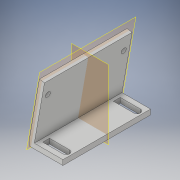
# Autodesk Inventor part: Part2
Saved by Autodesk Inventor 2019 (Build 230136000, 136)
## iProperties
Created: 2019-01-08
Part Number: Part2
Material: Generic
Document SubType Name: Modeling
Designer: Mataria
Density: 1 g/cm^3
Appearance: Default
Author: Mataria
Autodesk Inventor part; units mm, degrees
ref_plane "YZ Plane" through (0, 0, 0) normal (1, 0, 0) x (0, 1, 0)
ref_plane "XZ Plane" through (0, 0, 0) normal (0, 1, 0) x (-1, 0, 0)
ref_plane "XY Plane" through (0, 0, 0) normal (0, 0, 1) x (1, 0, 0)
sketch "Sketch1" plane through (0, 0, 0) normal (1, 0, 0) x (0, 1, 0)
  point P0 (0, 0)
sketch "Sketch2" plane through (0, 0, 0) normal (0, 0, 1) x (1, 0, 0)
  line L0 (0, 0) -> (20, 0)
  line L1 (20, 0) -> (20, 3)
  line L2 (0, 0) -> (0, 3)
  line L3 (0, 3) -> (6.0777, 37.4683)
  line L4 (0, 3) -> (35, 3) construction
  line L5 (6.0777, 37.4683) -> (9.0321, 36.9473)
  line L6 (9.0321, 36.9473) -> (3.0463, 3)
  line L7 (3.0463, 3) -> (20, 3)
  dimension "d0" = 20
  dimension "d1" = 3
  dimension "d2" = 3
  dimension "d4" = 35
  dimension "d5" = 80
  dimension "d6" = 3
  constraints: 16 end point, 2 horizontal, 2 perpendicular, 1 equal length, 1 point on line, 1 vertical
  measures "d0" distance of L0.start L0.end
  measures "d1" distance of L0.end L1.end
  measures "d2" distance of L0.start L2.end
  measures "d4" distance of L2.end L3.end
  measures "d5" angle of L4 L3
  measures "d6" distance of L3.end L5.end
extrude "Extrusion1" add sketch "Sketch2" along normal blind 26 and the other way blind 26
ref_plane "Work Plane1" through (7.5549, 37.2078, 26) normal (0.9848, -0.1736, 0) x (0, 0, -1)
ref_plane "Work Plane2" through (0, 0, 0) normal (0, 0, 1) x (1, 0, 0)
sketch "Sketch3" plane through (9.0321, 36.9473, 26) normal (0.9848, -0.1736, 0) x (0, 0, -1)
  point P0 (26, -37.9544)
sketch "Sketch4" plane through (9.0321, 36.9473, 26) normal (0.9848, -0.1736, 0) x (0, 0, -1)
  circle A0 centre (3.5, -8.527) radius 1.5
  circle A1 centre (48.5, -8.527) radius 1.5
  point P0 (26, -37.9544)
  dimension "d11" = 3
  dimension "d12" = 3
  constraints: 2 centre point
  measures "d11" diameter of A0
  measures "d12" diameter of A1
extrude "Extrusion2" cut sketch "Sketch4" against normal blind 3 contours A0
sketch "Sketch5" plane through (9.0321, 36.9473, 26) normal (0.9848, -0.1736, 0) x (0, 0, -1)
  circle A0 centre (48.5, -8.527) radius 1.5
  point P0 (26, -37.9544)
  dimension "d15" = 3
  constraints: 1 centre point
  measures "d15" diameter of A0
extrude "Extrusion3" cut sketch "Sketch5" against normal blind 3
sketch "Sketch6" plane through (3.0463, 3, 26) normal (0, 1, 0) x (1, 0, 0)
  point P0 (-3.0463, 26)
sketch "Sketch7" plane through (0, 0, 26) normal (0, -1, 0) x (1, 0, 0)
  line L0 (6.0777, -52) -> (6.0777, 0) projected
  line L1 (5, -3) -> (17, -3)
  line L2 (17, -7) -> (5, -7)
  arc A0 (17, -7) -> (17, -3) centre (17, -5) ccw
  line L3 (5, -3) -> (5, -7)
  ellipse E0 centre (4.597, -3.5) end of major axis (4.597, -2) minor radius 0.2605 projected
  line L4 (20, -52) -> (20, 0) projected
  line L5 (5, -49) -> (17, -49)
  line L6 (17, -45) -> (5, -45)
  arc A1 (17, -49) -> (17, -45) centre (17, -47) ccw
  line L7 (5, -49) -> (5, -45)
  point P0 (0, -26)
  dimension "d19" = 12
  constraints: 12 end point, 4 point on circle, 2 centre point, 1 horizontal, 1 perpendicular, 1 vertical, 1 other
  measures "d19" distance of L1.start L1.end
extrude "Extrusion4" cut sketch "Sketch7" against normal blind 3 contours L5 L7 L6 L0 | L2 L3 L1 L0 | L0 L1 A0 L2 | L0 L6 A1 L5
body "Solid1"
